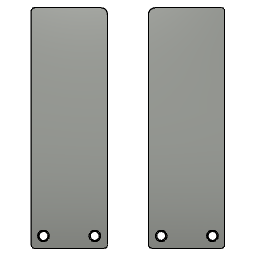
mriya-cnc-mcu-cover-v1.00 (Autodesk Fusion 360 design; units mm, degrees)
Autodesk Fusion 360 part; units mm, degrees
sketch "mriya-mcu-cover" plane through (0, 0, 0) normal (0, 0, 1) x (1, 0, 0)
  circle A0 centre (-20.6, 8) radius 1.1
  circle A1 centre (-8.1, 8) radius 1.1
  circle A2 centre (-20.6, 8) radius 1.4
  circle A3 centre (-8.1, 8) radius 1.4
  line L0 (-21.45, 24.8) -> (-21.45, 60.1)
  line L1 (-8.45, 23.7) -> (-20.35, 23.7)
  line L2 (-9.15, 27.5) -> (-19.65, 27.5) construction
  line L3 (-19.65, 55) -> (-9.15, 55) construction
  line L4 (-8.45, 61.2) -> (-20.35, 61.2)
  line L5 (-20.65, 54) -> (-20.65, 28.5) construction
  line L6 (-8.15, 28.5) -> (-8.15, 54) construction
  line L7 (-7.35, 60.1) -> (-7.35, 24.8)
  line L8 (-23.6, 5.8) -> (-23.6, 62.7) construction
  line L9 (-6.6, 63.6) -> (-22.8, 63.6)
  line L10 (-5, 62) -> (-5, 5.8)
  line L11 (-22.8, 5) -> (-5.9, 5) construction
  line L12 (-5.1, 62) -> (-5.1, 5.8) construction
  line L13 (-6.6, 63.5) -> (-22.8, 63.5) construction
  arc A4 (-5.1, 62) -> (-6.6, 63.5) centre (-6.6, 62) ccw construction
  arc A5 (-22.8, 63.5) -> (-23.6, 62.7) centre (-22.8, 62.7) ccw construction
  arc A6 (-23.6, 5.8) -> (-22.8, 5) centre (-22.8, 5.8) ccw construction
  arc A7 (-5.9, 5) -> (-5.1, 5.8) centre (-5.9, 5.8) ccw construction
  line L14 (-5.8, 5) -> (-22.8, 5)
  line L15 (-23.6, 5.8) -> (-23.6, 62.8)
  arc A8 (-22.8, 63.6) -> (-23.6, 62.8) centre (-22.8, 62.8) ccw
  arc A9 (-5, 62) -> (-6.6, 63.6) centre (-6.6, 62) ccw
  arc A10 (-5.8, 5) -> (-5, 5.8) centre (-5.8, 5.8) ccw
  arc A11 (-23.6, 5.8) -> (-22.8, 5) centre (-22.8, 5.8) ccw
  arc A12 (-19.65, 55) -> (-20.65, 54) centre (-19.65, 54) ccw construction
  arc A13 (-8.15, 54) -> (-9.15, 55) centre (-9.15, 54) ccw construction
  arc A14 (-20.65, 28.5) -> (-19.65, 27.5) centre (-19.65, 28.5) ccw construction
  arc A15 (-9.15, 27.5) -> (-8.15, 28.5) centre (-9.15, 28.5) ccw construction
  arc A16 (-21.45, 24.8) -> (-20.35, 23.7) centre (-20.35, 24.8) ccw
  arc A17 (-8.45, 23.7) -> (-7.35, 24.8) centre (-8.45, 24.8) ccw
  line L16 (-5.7, 26.1) -> (-5.7, 62) construction
  line L17 (-18.5, 62.9) -> (-6.6, 62.9) construction
  arc A18 (-19.1, 63.5) -> (-18.5, 62.9) centre (-18.5, 63.5) ccw construction
  arc A19 (-5.7, 26.1) -> (-5.1, 25.5) centre (-5.1, 26.1) ccw construction
  arc A20 (-5.7, 62) -> (-6.6, 62.9) centre (-6.6, 62) ccw construction
  circle A21 centre (-14.4, 14.5) radius 5 construction
  circle A22 centre (-20.6, 20.5) radius 1.7 construction
  circle A23 centre (-8.1, 20.5) radius 1.7 construction
  arc A24 (-20.35, 61.2) -> (-21.45, 60.1) centre (-20.35, 60.1) ccw
  arc A25 (-7.35, 60.1) -> (-8.45, 61.2) centre (-8.45, 60.1) ccw
  dimension "d8" = 2.2
  dimension "d9" = 2.2
  dimension "d17" = 2.8
  dimension "d18" = 2.8
  dimension "d585" = 10
  dimension "d588" = 3.4
  dimension "d589" = 3.4
  constraint concentric A1 A3
  constraint perpendicular L1 L7
  constraint perpendicular L2 L5
  constraint vertical L5
  constraint perpendicular L3 L5
  constraint vertical L6
  constraint perpendicular L8 L9
  constraint horizontal L11
  constraint perpendicular L8 L11
  constraint tangent L13 A4
  constraint tangent L12 A4
  constraint tangent L13 A5
  constraint tangent L8 A5
  constraint tangent L8 A6
  constraint tangent L11 A6
  constraint tangent L12 A7
  constraint tangent L11 A7
  constraint perpendicular L10 L14
  constraint perpendicular L9 L15
  constraint tangent L9 A8
  constraint tangent L15 A8
  constraint tangent L9 A9
  constraint tangent L10 A9
  constraint tangent L14 A10
  constraint tangent L10 A10
  constraint tangent L15 A11
  constraint tangent L14 A11
  constraint tangent L3 A12
  constraint tangent L5 A12
  constraint tangent L3 A13
  constraint tangent L6 A13
  constraint tangent L5 A14
  constraint tangent L2 A14
  constraint tangent L6 A15
  constraint tangent L2 A15
  constraint tangent L0 A16
  constraint tangent L1 A16
  constraint tangent L7 A17
  constraint tangent L1 A17
  constraint tangent L17 A18
  constraint tangent L16 A19
  constraint tangent L17 A20
  constraint tangent L16 A20
  constraint tangent L0 A24
  constraint tangent L4 A24
  constraint tangent L4 A25
  constraint tangent L7 A25
  measures "d8" diameter of A0
  measures "d9" diameter of A1
  measures "d17" diameter of A2
  measures "d18" diameter of A3
  measures "d585" diameter of A21
  measures "d588" diameter of A22
  measures "d589" diameter of A23
extrude "Extrude75" add sketch "mriya-mcu-cover" along normal blind 1.5 contours L0 L1 L4 L7 A16 A17 A24 A25 | L9 L10 L14 L15 A8 A9 A10 A11 makes body 1
extrude "Extrude77" add sketch "mriya-mcu-cover" along normal blind 0.7 contours A2 | A3 bodies 1
mirror "Mirror9" about plane through (0, 0, 0) normal (1, 0, 0) of bodies 1 makes body 2
named bodies: "Right", "Left"
